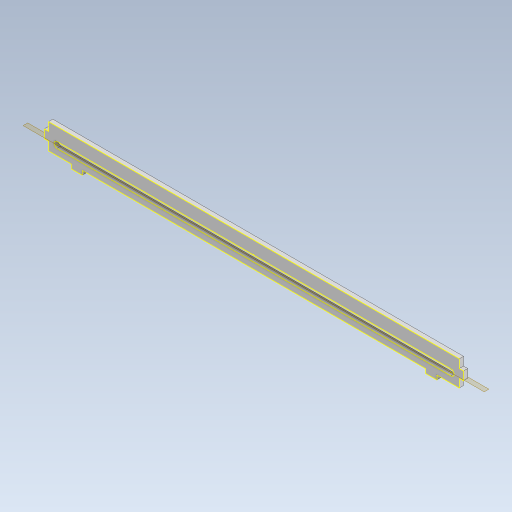
# Autodesk Inventor part: 零件4
Saved by Autodesk Inventor 2023 (Build 270158000, 158)
## iProperties
Created: 2023-04-16
Part Number: 零件4
Material: 一般
Document SubType Name: Modeling
Designer: JOU
Density: 1 g/cm^3
Appearance: 預設
Author: JOU
Autodesk Inventor part; units mm, degrees
ref_plane "YZ Plane" through (0, 0, 0) normal (1, 0, 0) x (0, 1, 0)
ref_plane "XZ Plane" through (0, 0, 0) normal (0, 1, 0) x (-1, 0, 0)
ref_plane "XY Plane" through (0, 0, 0) normal (0, 0, 1) x (1, 0, 0)
sketch "草圖1" plane through (0, 0, 0) normal (0, 0, 1) x (1, 0, 0)
  line L0 (-140, 0) -> (140, 0) construction
  line L1 (-140, 0) -> (140, 0) construction
  line L2 (-140, -9) -> (140, -9)
  line L3 (140, 9) -> (-140, 9)
  arc A0 (-140, 9) -> (-140, -9) centre (-140, 0) ccw
  arc A1 (140, -9) -> (140, 9) centre (140, 0) ccw
  line L4 (-140, -2.35) -> (140, -2.35) construction
  line L5 (-140, -4.5) -> (140, -4.5)
  line L6 (140, -0.2) -> (-140, -0.2)
  arc A2 (-140, -0.2) -> (-140, -4.5) centre (-140, -2.35) ccw
  arc A3 (140, -4.5) -> (140, -0.2) centre (140, -2.35) ccw
  line L7 (140, -2.35) -> (140, 0) construction
  line L8 (-140, 9) -> (-149, 9)
  line L9 (-149, 9) -> (-149, -9)
  line L10 (-149, -9) -> (-140, -9)
  line L11 (-140, -9) -> (-140, 9)
  line L12 (140, 9) -> (149, 9)
  line L13 (149, 9) -> (149, -9)
  line L14 (149, -9) -> (140, -9)
  line L15 (140, -9) -> (140, 9)
  point P0 (0, 0)
  point P1 (0, 0)
  point P2 (0, 0)
  point P3 (0, -2.35)
  point P4 (149, 0)
  point P5 (-140, -9)
  point P6 (-149, 0)
  dimension "d5" = 9
  dimension "d7" = 280
  dimension "d22" = 2.15
  dimension "d24" = 4.5
  constraints: 38 end point, 11 tangent, 8 parallel, 8 point on circle, 4 centre point, 3 horizontal, 3 midpoint, 3 point on line, 2 coincident, 2 perpendicular, 1 vertical, 1 vertical alignment
  measures "d5" radius of A0
  measures "d7" distance of L1.end L1.start
  measures "d22" radius of A3
  measures "d24" distance between parallel lines of L2 L5
extrude "擠出1" add sketch "草圖1" along normal blind 3 contours L11 L5 L15 L2 | L10 L9 A0 | A0 L11 A2 | L15 A3 A1 | A1 L13 L14 | L9 L8 A0 | A1 L12 L13 | L3 L15 L6 L11
sketch "草圖2" plane through (0, 0, 3) normal (0, 0, 1) x (1, 0, 0)
  line L0 (-208.6, 0) -> (208.6, 0) projected
  line L1 (-130, -9) -> (-122, -9)
  line L2 (-122, -9) -> (-122, -12)
  line L3 (-122, -12) -> (-130, -12)
  line L4 (-130, -12) -> (-130, -9)
  line L5 (122, -9) -> (130, -9)
  line L6 (130, -9) -> (130, -12)
  line L7 (130, -12) -> (122, -12)
  line L8 (122, -12) -> (122, -9)
  arc A0 (-140, -0.2) -> (-140, -4.5) centre (-140, -2.35) ccw projected
  arc A1 (140, -4.5) -> (140, -0.2) centre (140, -2.35) ccw projected
  line L9 (-149, -9) -> (149, -9) projected
  point P0 (0, 0)
  point P1 (130, -10.5)
  point P2 (-130, -10.5)
  dimension "d17" = 8
  dimension "d18" = 3
  dimension "d19" = 3
  dimension "d20" = 8
  dimension "d25" = 10
  dimension "d26" = 10
  constraints: 16 end point, 5 perpendicular, 2 collinear, 2 midpoint, 1 parallel
  measures "d17" distance of L2.end L3.end
  measures "d18" distance of L1.end L2.end
  measures "d19" distance of L5.end L6.end
  measures "d20" distance of L6.end L7.end
  measures "d25" horizontal distance of A1.centre point (130, -10.5)
  measures "d26" horizontal distance of point (-130, -10.5) A0.centre
extrude "擠出2" add sketch "草圖2" against normal up to surface (3 mm away)
ref_plane "工作平面2" through (-140, -2.35, 0) normal (0, 1, 0) x (1, 0, 0)
sketch "草圖4" plane through (0, 0, 3) normal (0, 0, 1) x (1, 0, 0)
  line L0 (149, 9) -> (-149, 9) projected
  line L1 (-149, -9) -> (-130, -9) projected
  line L2 (-149, 9) -> (-146, 9)
  line L3 (-146, 9) -> (-146, -9)
  line L4 (-146, -9) -> (-149, -9)
  line L5 (-149, -9) -> (-149, 9)
  line L6 (-149, 9) -> (-149, -9) projected
  line L7 (-149, 3) -> (-146, 3)
  line L8 (-146, 3) -> (-146, -3)
  line L9 (-146, -3) -> (-149, -3)
  line L10 (-149, -3) -> (-149, 3)
  line L11 (149, -9) -> (149, 9) projected
  line L12 (149, -9) -> (146, -9)
  line L13 (146, -9) -> (146, 9)
  line L14 (146, 9) -> (149, 9)
  line L15 (149, 9) -> (149, -9)
  line L16 (149, -3) -> (146, -3)
  line L17 (146, -3) -> (146, 3)
  line L18 (146, 3) -> (149, 3)
  line L19 (149, 3) -> (149, -3)
  point P0 (0, 0)
  dimension "d27" = 6
  dimension "d28" = 6
  dimension "d29" = 3
  dimension "d32" = 3
  constraints: 32 end point, 8 parallel, 6 point on line, 4 horizontal, 4 perpendicular, 2 collinear
  measures "d27" distance between parallel lines of L9 L7
  measures "d28" distance between parallel lines of L0 L7
  measures "d29" distance between parallel lines of L5 L3
  measures "d32" distance of L11.start L12.end
extrude "擠出3" cut sketch "草圖4" against normal up to surface (3 mm away) contours L11 L18 L13 L0 | L3 L7 L5 L0 | L11 L12 L13 L16 | L3 L1 L5 L9
sketch "草圖5" plane through (0, 0, 3) normal (0, 0, 1) x (1, 0, 0)
  arc A0 (-140, -0.2) -> (-140, -4.5) centre (-140, -2.35) ccw projected
  line L0 (-140, -0.2) -> (140, -0.2) projected
  arc A1 (140, -4.5) -> (140, -0.2) centre (140, -2.35) ccw projected
  line L1 (140, -4.5) -> (-140, -4.5) projected
  line L2 (-146, 9) -> (-146, 3) projected
  line L3 (-146, 3) -> (-149, 3) projected
  line L4 (-149, 3) -> (-149, -3) projected
  line L5 (-149, -3) -> (-146, -3) projected
  line L6 (-146, -3) -> (-146, -9) projected
  line L7 (-146, -9) -> (-130, -9) projected
  line L8 (-130, -9) -> (-130, -12) projected
  line L9 (-130, -12) -> (-122, -12) projected
  line L10 (-122, -12) -> (-122, -9) projected
  line L11 (-122, -9) -> (122, -9) projected
  line L12 (122, -9) -> (122, -12) projected
  line L13 (122, -12) -> (130, -12) projected
  line L14 (130, -12) -> (130, -9) projected
  line L15 (130, -9) -> (146, -9) projected
  line L16 (146, -9) -> (146, -3) projected
  line L17 (146, -3) -> (149, -3) projected
  line L18 (149, -3) -> (149, 3) projected
  line L19 (149, 3) -> (146, 3) projected
  line L20 (146, 3) -> (146, 9) projected
  line L21 (146, 9) -> (-146, 9) projected
  point P0 (0, 0)
equation "\"d32\" = d29"
